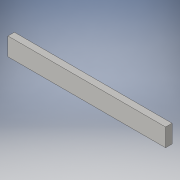
# Autodesk Inventor part: Part10
Saved by Autodesk Inventor 2016 (Build 200138000, 138)
## iProperties
Created: 2016-01-16
Part Number: Part10
Material: Generic
Document SubType Name: Modeling
Designer: Thariq
Density: 1 g/cm^3
Appearance: Default
Author: Thariq
Autodesk Inventor part; units mm, degrees
ref_plane "YZ Plane" through (0, 0, 0) normal (1, 0, 0) x (0, 1, 0)
ref_plane "XZ Plane" through (0, 0, 0) normal (0, 1, 0) x (-1, 0, 0)
ref_plane "XY Plane" through (0, 0, 0) normal (0, 0, 1) x (1, 0, 0)
sketch "Sketch1" plane through (0, 0, 0) normal (0, 1, 0) x (-1, 0, 0)
  line L0 (56.4266, 74.8912) -> (-54.7876, 74.8912)
  line L1 (-54.7876, 74.8912) -> (-54.7876, 70.4883)
  line L2 (-54.7876, 70.4883) -> (56.4266, 70.4883)
  line L3 (56.4266, 70.4883) -> (56.4266, 74.8912)
  line L4 (56.4266, -41.3782) -> (-54.7876, -41.3782)
  line L5 (-54.7876, -41.3782) -> (-54.7876, -45.9442)
  line L6 (-54.7876, -45.9442) -> (56.4266, -45.9442)
  line L7 (56.4266, -45.9442) -> (56.4266, -41.3782)
  point P0 (0, 0)
  constraints: 16 end point, 4 parallel, 2 horizontal, 2 perpendicular, 2 point on line
extrude "Extrusion1" add sketch "Sketch1" along normal blind 12.7 contours L7 L6 L5 L4
body "Solid1"
